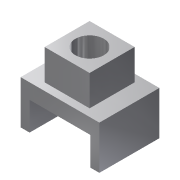
# Autodesk Inventor part: suporte-barra
Saved by Autodesk Inventor 2015 (Build 190159000, 159)
## iProperties
Created: 2016-08-11
Part Number: suporte-barra
Material: Steel, Carbon
Document SubType Name: Modeling
Designer: EriveltonDell
Density: 7.87 g/cm^3
Appearance: Aluminum - Polished
Mass: 377.778 g
Surface Area: 137.801 cm^2
Volume: 48.0022 cm^3
Author: EriveltonDell
Autodesk Inventor part; units mm, degrees
ref_plane "YZ Plane" through (0, 0, 0) normal (1, 0, 0) x (0, 1, 0)
ref_plane "XZ Plane" through (0, 0, 0) normal (0, 1, 0) x (-1, 0, 0)
ref_plane "XY Plane" through (0, 0, 0) normal (0, 0, 1) x (1, 0, 0)
sketch "Sketch1" plane through (0, 0, 0) normal (0, 1, 0) x (-1, 0, 0)
  line L0 (20, -0.25) -> (20, 20)
  line L1 (20, 20) -> (-20.5, 20)
  line L2 (-20.5, 20) -> (-20.5, -0.25)
  line L3 (20, 9.875) -> (-20.5, 9.875)
  dimension "d49" = 40.5
  constraints: 8 end point, 2 midpoint, 2 perpendicular
  measures "d49" distance of L0.end L1.end
extrude "Extrusion1" add sketch "Sketch1" along normal mid plane 40
sketch "Sketch6" plane through (0, 0, 0) normal (0, 0, 1) x (1, 0, 0)
  line L0 (0, 0) -> (-15, 0)
  line L1 (-15, 0) -> (-15, -15)
  line L2 (-15, -15) -> (15, -15)
  line L3 (15, -15) -> (15, 15)
  line L4 (15, 15) -> (-15, 15)
  line L5 (-15, 15) -> (-15, 0)
  dimension "d64" = 15
  dimension "d65" = 15
  dimension "d66" = 90
  dimension "d67" = 30
  dimension "d68" = 90
  dimension "d69" = 30
  dimension "d70" = 90
  dimension "d71" = 30
  dimension "d72" = 90
  constraints: 12 end point, 4 perpendicular, 1 coincident, 1 horizontal
  measures "d64" distance of L0.start L0.end
  measures "d65" distance of L0.end L1.end
  measures "d66" angle of L1 L0
  measures "d67" distance of L1.end L2.end
  measures "d68" angle of L2 L1
  measures "d69" distance of L2.end L3.end
  measures "d70" angle of L3 L2
  measures "d71" distance of L3.end L4.end
  measures "d72" angle of L4 L3
extrude "Extrusion6" add sketch "Sketch6" along normal blind 40.4
hole "Hole2" at (0, 0, 40.4) direction (0, 0, -1) diameter 19 depth 15
fillet "Fillet3" [suppressed]
sketch "Sketch8" plane through (0, 0, 0) normal (0, 0, -1) x (-1, 0, 0)
  line L0 (15, -15) -> (-15, -15)
  line L1 (-15, -15) -> (-15, 15)
  line L2 (-15, 15) -> (15, 15)
  line L3 (15, 15) -> (15, -15)
  point P0 (0, 0)
  constraints: 8 end point, 2 parallel, 1 horizontal, 1 perpendicular
extrude "Extrusion8" cut sketch "Sketch8" against normal blind 10
sketch "Sketch10" plane through (-20, 20, 20) normal (0, 0, 1) x (1, 0, 0)
  line L0 (0, 0) -> (-6, 0)
  line L1 (-6, 0) -> (-6, -40)
  line L2 (-6, -40) -> (0, -40)
  line L3 (0, -40) -> (0, 0)
  line L4 (40.5, 0) -> (46.5, 0)
  line L5 (46.5, 0) -> (46.5, -40)
  line L6 (46.5, -40) -> (40.5, -40)
  line L7 (40.5, -40) -> (40.5, 0)
  point P0 (20, -20)
  dimension "d73" = 6
  dimension "d74" = 6
  dimension "d75" = 40.5
  constraints: 16 end point, 4 parallel, 2 horizontal, 2 perpendicular, 1 point on line
  measures "d73" distance of L5.end L6.end
  measures "d74" distance of L1.end L2.end
  measures "d75" distance between parallel lines of L7 L3
extrude "Extrusion9" add sketch "Sketch10" against normal blind 29
body "Solid1"
